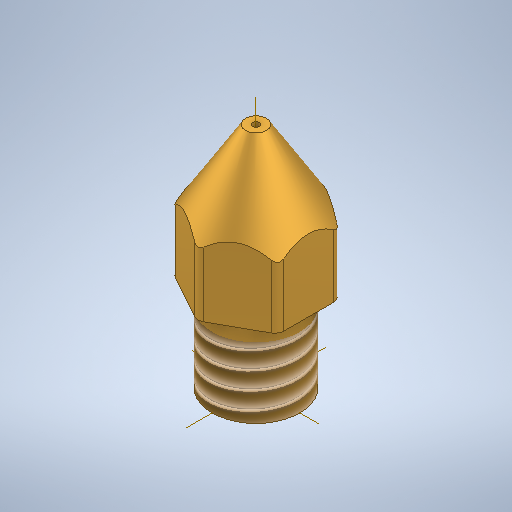
# Autodesk Inventor part: Nozzle 0.4mm
Saved by Autodesk Inventor 2025 (Build 290162000, 162)
## iProperties
Created: 2025-02-05
Part Number: Nozzle 0.4mm
Material: Brass, Soft Yellow
Document SubType Name: Modeling
Designer: MAL16204
Density: 8.47 g/cm^3
Appearance: Brass - Satin
Author: MAL16204
Autodesk Inventor part; units mm, degrees
ref_plane "YZ Plane" through (0, 0, 0) normal (1, 0, 0) x (0, 1, 0)
ref_plane "XZ Plane" through (0, 0, 0) normal (0, 1, 0) x (-1, 0, 0)
ref_plane "XY Plane" through (0, 0, 0) normal (0, 0, 1) x (1, 0, 0)
sketch "Sketch1" plane through (0, 0, 0) normal (0, 1, 0) x (-1, 0, 0)
  line L0 (0, -4.739) -> (0, 4.739) construction
  line L1 (4.2, 0) -> (-4.2, 0) construction
  line L2 (3, 1.7164) -> (3, -1.7164)
  line L3 (3, -1.7164) -> (0, -3.385)
  line L4 (0, -3.385) -> (-3, -1.7164)
  line L5 (-3, -1.7164) -> (-3, 1.7164)
  line L6 (-3, 1.7164) -> (0, 3.385)
  line L7 (0, 3.385) -> (3, 1.7164)
  point P0 (3, 0)
  point P1 (-3, 0)
  dimension "d2" = 6.77
  dimension "d3" = 6
  constraints: 12 end point, 5 equal length, 3 point on line, 2 midpoint, 1 parallel, 1 vertical
  measures "d2" distance of L3.end L6.end
  measures "d3" distance between parallel lines of L5 L2
extrude "Extrusion1" add sketch "Sketch1" along normal blind 13
fillet "Fillet1" radius 0.5 6 edges at (0, 6.5, 3.385) (3, 6.5, 1.7164) (3, 6.5, -1.7164) (0, 6.5, -3.385) (-3, 6.5, -1.7164) (-3, 6.5, 1.7164)
sketch "Sketch2" plane through (0, 0, 0) normal (0, 0, 1) x (1, 0, 0)
  line L0 (-0.243, 13) -> (0.243, 13) projected
  line L1 (0, 13) -> (-0.1, 13)
  line L2 (-0.1, 13) -> (-0.6, 13)
  line L3 (-0.6, 13) -> (-3, 9.0992)
  line L4 (-0.243, 13) -> (-2.743, 13) projected
  line L5 (0, 13) -> (0, 13.665)
  line L6 (-0.6, 13) -> (-4.1, 13)
  line L7 (-4.1, 13) -> (-4.1, 7.3113)
  line L8 (-3, 13) -> (-3, 0) projected
  line L9 (-4.1, 7.3113) -> (-3, 9.0992)
  point P0 (0, 0)
  dimension "d7" = 0.1
  dimension "d8" = 0.5
  dimension "d9" = 4.58
  dimension "d11" = 3.5
  constraints: 14 end point, 2 point on line, 2 vertical, 1 collinear, 1 midpoint
  measures "d7" distance of L1.start L1.end
  measures "d8" distance of L1.end L2.end
  measures "d9" distance of L2.end L3.end
  measures "d11" distance of L2.end L6.end
revolve "Revolution1" cut sketch "Sketch2" angle 360 about axis through (0, 13, 0) along (0, 1, 0)
sketch "Sketch3" plane through (0, 0, 0) normal (0, -1, 0) x (1, 0, 0)
  circle A0 centre (0, 0) radius 2.5
  arc A1 (-2.743, 1.8593) -> (-3, 1.4224) centre (-2.5, 1.4224) ccw projected
  line L0 (-3, -1.4224) -> (-3, 1.4224) projected
  arc A2 (-3, -1.4224) -> (-2.743, -1.8593) centre (-2.5, -1.4224) ccw projected
  line L1 (-0.243, -3.2498) -> (-2.743, -1.8593) projected
  arc A3 (-0.243, -3.2498) -> (0.243, -3.2498) centre (0, -2.8129) ccw projected
  line L2 (2.743, -1.8593) -> (0.243, -3.2498) projected
  arc A4 (2.743, -1.8593) -> (3, -1.4224) centre (2.5, -1.4224) ccw projected
  line L3 (3, 1.4224) -> (3, -1.4224) projected
  arc A5 (3, 1.4224) -> (2.743, 1.8593) centre (2.5, 1.4224) ccw projected
  line L4 (0.243, 3.2498) -> (2.743, 1.8593) projected
  arc A6 (0.243, 3.2498) -> (-0.243, 3.2498) centre (0, 2.8129) ccw projected
  line L5 (-2.743, 1.8593) -> (-0.243, 3.2498) projected
  dimension "d12" = 5
  constraints: 1 centre point, 1 coincident
  measures "d12" diameter of A0
extrude "Extrusion2" cut sketch "Sketch3" against normal blind 5
thread "Thread1" size "M6x1" class "6g" standard "ANSI Metric M Profile" length 4
sketch "Sketch4" plane through (0, 0, 0) normal (0, -1, 0) x (1, 0, 0)
  circle A0 centre (0, 0) radius 0.6 projected
  circle A1 centre (0, 0) radius 1
  point P0 (0, 0)
  dimension "d20" = 2
  constraints: 1 centre point, 1 coincident
  measures "d20" diameter of A1
extrude "Extrusion3" cut sketch "Sketch4" against normal blind 11 contours A0 | A1
sketch "Sketch5" plane through (0, 0, 0) normal (0, 0, 1) x (1, 0, 0)
  line L0 (1, 11) -> (-1, 11) projected
  line L1 (-1, 11) -> (-0.2, 12.51)
  line L2 (1, 11) -> (0.2, 12.51)
  line L3 (-0.2, 12.51) -> (0.2, 12.51) construction
  line L4 (0, -2.6) -> (0, 15.6) projected
  line L5 (0.6, 13) -> (-0.6, 13) projected
  line L6 (0.2, 12.51) -> (0.2, 13.1094)
  line L7 (0.2, 13.1094) -> (-0.2, 13.1094)
  line L8 (-0.2, 13.1094) -> (-0.2, 12.51)
  point P0 (0, 0)
  point P1 (0, 12.51)
  point P2 (0, 13.1094)
  point P3 (0, 11)
  dimension "d25" = 0.4
  dimension "d26" = 1.51
  constraints: 12 end point, 1 equal length, 1 horizontal, 1 midpoint, 1 parallel, 1 point on line, 1 vertical
  measures "d25" distance of L1.end L2.end
  measures "d26" distance between parallel lines of L0 L3
revolve "Revolution2" cut sketch "Sketch5" angle 360 about axis through (0, -10, 0) along (0, 1, 0) contours L0 L4 L5 L6 L2 | L4 L7 L6 L5
body "Solid1"
